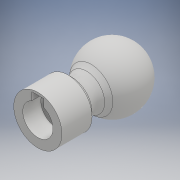
# Autodesk Inventor part: 伸縮缸 球軸 球
Saved by Autodesk Inventor 2017 (Build 210142000, 142)
## iProperties
Part Number: 伸縮缸 球軸 球
Material: 一般
Document SubType Name: Modeling
Designer: NB23-1
Density: 1 g/cm^3
Appearance: 預設
Author: NB23-1
Autodesk Inventor part; units mm, degrees
note: some values were not read from the file. Chosen so that the rebuilt part matches the saved one: edges of "圓角2".
ref_plane "YZ Plane" through (0, 0, 0) normal (1, 0, 0) x (0, 1, 0)
ref_plane "XZ Plane" through (0, 0, 0) normal (0, 1, 0) x (-1, 0, 0)
ref_plane "XY Plane" through (0, 0, 0) normal (0, 0, 1) x (1, 0, 0)
sketch "草圖1" plane through (0, 0, 0) normal (0, 1, 0) x (-1, 0, 0)
  circle A0 centre (0, 0) radius 4
  dimension "d0" = 8
  constraints: 1 centre point, 1 coincident
  measures "d0" diameter of A0
extrude "擠出1" add sketch "草圖1" along normal blind 5
sketch "草圖2" plane through (0, 0, 0) normal (0, -1, 0) x (1, 0, 0)
  circle A0 centre (0, 0) radius 2.5
  dimension "d3" = 5
  constraints: 1 centre point, 1 coincident
  measures "d3" diameter of A0
extrude "擠出2" cut sketch "草圖2" against normal blind 3
sketch "草圖3" plane through (0, 5, 0) normal (0, 1, 0) x (1, 0, 0)
  circle A0 centre (0, 0) radius 2.5
  dimension "d6" = 5
  constraints: 1 centre point, 1 coincident
  measures "d6" diameter of A0
extrude "擠出3" add sketch "草圖3" along normal blind 3
chamfer "倒角1" distance 1.5 angle 45 1 edges at (-2.5, 5, 0)
sketch "草圖4" plane through (0, 0, 0) normal (0, 0, 1) x (1, 0, 0)
  arc A0 (0, 7.3301) -> (0, 17.3301) centre (0, 12.3301) ccw
  line L0 (0, 12.3301) -> (0, 17.3301) construction
  line L1 (0, 12.3301) -> (0, 7.3301) construction
  line L2 (0, 17.3301) -> (0, 7.3301)
  line L3 (2.5, 8) -> (-2.5, 8) projected
  point P0 (0, 0)
  dimension "d12" = 5
  dimension "d13" = 180
  dimension "d14" = 90
  dimension "d15" = 2.5
  constraints: 6 end point, 3 point on circle, 1 centre point
  measures "d12" radius of A0
  measures "d13" angle of L1 L0
  measures "d14" angle of L3 L1
  measures "d15" distance from line of L3.start L1
revolve "迴轉1" add sketch "草圖4" angle 360 about axis through (0, 12.3301, 0) along (0, -1, 0)
fillet "圓角1" radius 4 1 edges at (-2.5, 8, 0)
sketch "草圖6" plane through (0, 0, 0) normal (0, -1, 0) x (1, 0, 0)
  circle A0 centre (0, 0) radius 2.5 projected
  line L0 (-1, 2.2913) -> (1, 2.2913)
  line L1 (1, 2.2913) -> (1, 3.5913)
  line L2 (1, 3.5913) -> (-1, 3.5913)
  line L3 (-1, 3.5913) -> (-1, 2.2913)
  dimension "d20" = 2
  dimension "d21" = 1.3
  constraints: 8 end point, 2 parallel, 2 point on circle, 1 horizontal, 1 perpendicular
  measures "d20" distance of L1.end L2.end
  measures "d21" distance of L0.end L1.end
extrude "擠出5" cut sketch "草圖6" against normal blind 3 contours A0 L3 L2 L1
fillet "圓角2" radius 2 1 edges at (-2.5, 6.4999, 0)
sketch "草圖5" plane through (0, 0, 0) normal (0, -1, 0) x (1, 0, 0)
  circle A0 centre (0, 0) radius 3.2143 projected
  circle A1 centre (0, 0) radius 2.5 projected
  circle A2 centre (0, 0) radius 4 projected
